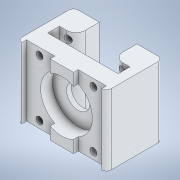
# Autodesk Inventor part: Tensor
Saved by Autodesk Inventor 2021 (Build 250183000, 183)
## iProperties
Created: 2022-10-27
Part Number: Tensor
Material: Generic
Document SubType Name: Modeling
Designer: USUARIO
Density: 1 g/cm^3
Appearance: White
Author: USUARIO
Autodesk Inventor part; units mm, degrees
ref_plane "YZ Plane" through (0, 0, 0) normal (1, 0, 0) x (0, 1, 0)
ref_plane "XZ Plane" through (0, 0, 0) normal (0, 1, 0) x (-1, 0, 0)
ref_plane "XY Plane" through (0, 0, 0) normal (0, 0, 1) x (1, 0, 0)
sketch "Sketch1" plane through (0, 0, 0) normal (0, 1, 0) x (-1, 0, 0)
  line L0 (0, -37.4557) -> (0, 23.9689) construction
  line L1 (8, -2) -> (8, -12)
  line L2 (8, -12) -> (19, -12)
  line L3 (19, -12) -> (19, 12)
  line L4 (19, 12) -> (2, 12)
  line L5 (8, -2) -> (15, -2)
  line L6 (15, -2) -> (15, 3)
  line L7 (15, 3) -> (0, 3)
  line L8 (0, -49.7407) -> (0, 36.2538) projected
  line L9 (-8, -2) -> (-8, -12)
  line L10 (-8, -12) -> (-19, -12)
  line L11 (-19, -12) -> (-19, 12)
  line L12 (-19, 12) -> (2, 12)
  line L13 (-8, -2) -> (-15, -2)
  line L14 (-15, -2) -> (-15, 3)
  line L15 (-15, 3) -> (0, 3)
  line L16 (26.6, 0) -> (-26.6, 0) projected
  point P0 (19, 0)
  point P1 (-19, 0)
  dimension "d12" = 15
  dimension "d13" = 5
  dimension "d14" = 7
  dimension "d15" = 10
  dimension "d16" = 11
  dimension "d18" = 9
  dimension "d19" = 17
  constraints: 30 end point, 7 symmetric about line, 3 parallel, 2 perpendicular, 2 point on line, 2 vertical, 1 collinear, 1 horizontal, 1 midpoint
  measures "d12" distance of L6.end L7.end
  measures "d13" distance of L5.end L6.end
  measures "d14" distance of L1.start L5.end
  measures "d15" distance of L1.start L1.end
  measures "d16" distance of L1.end L2.end
  measures "d18" distance between parallel lines of L4 L7
  measures "d19" distance of L3.end L4.end
extrude "Extrusion1" add sketch "Sketch1" along normal blind 30 contours L5 L6 L16 L3 L2 L1 | L6 L7 L8 L12 L4 L3 L16 | L15 L14 L16 L11 L12 L8 | L14 L13 L9 L10 L11 L16
fillet "Fillet1" radius 4 2 edges at (-8, 15, -2) (8, 15, -2)
sketch "Sketch2" plane through (-19, 0, 12) normal (0, 0, 1) x (1, 0, 0)
  line L0 (0, 0) -> (38, 0) projected
  line L1 (38, 0) -> (38, 30) projected
  line L2 (0, 30) -> (38, 30) projected
  line L3 (0, 0) -> (0, 30) projected
  line L4 (38, 0) -> (38, 30) projected
  line L5 (38, 15) -> (0, 15) construction
  line L6 (0, 0) -> (0, 30) projected
  circle A0 centre (19, 15) radius 11
  circle A1 centre (19, 15) radius 5
  line L7 (0, 0) -> (38, 0) projected
  line L8 (7, 30) -> (7, 0) projected
  line L9 (4, 30) -> (7, 30) projected
  line L10 (4, 0) -> (4, 30) projected
  line L11 (4, 0) -> (7, 0) projected
  line L12 (31, 0) -> (31, 30) projected
  line L13 (31, 0) -> (34, 0) projected
  line L14 (34, 0) -> (34, 30) projected
  line L15 (31, 30) -> (34, 30) projected
  circle A2 centre (30.5, 27) radius 1.5
  line L16 (19, 15) -> (19, 38.5815) construction
  circle A3 centre (7.5, 27) radius 1.5
  circle A4 centre (30.5, 3) radius 1.5
  circle A5 centre (7.5, 3) radius 1.5
  point P0 (19, 0)
  dimension "d23" = 22
  dimension "d24" = 10
  dimension "d25" = 3
  dimension "d26" = 11.5
  dimension "d27" = 12
  constraints: 6 centre point, 4 end point, 3 midpoint, 3 symmetric about line, 1 coincident, 1 vertical, 3 other
  measures "d23" diameter of A0
  measures "d24" diameter of A1
  measures "d25" diameter of A2
  measures "d26" horizontal distance of A0.centre A2.centre
  measures "d27" vertical distance of A2.centre A0.centre
extrude "Extrusion2" cut sketch "Sketch2" against normal blind 7 contours A0
extrude "Extrusion3" cut sketch "Sketch2" against normal through all contours A5 L8 | L8 A5 | A4 L12 | L12 A4 | A3 L8 | L8 A3 | A2 L12 | L12 A2 | A1
fillet "Fillet2" radius 2 4 edges at (19, 15, 12) (-19, 15, 12) (-19, 15, -12) (19, 15, -12)
sketch "Boceto4" plane through (-17, 0, 12) normal (0, 0, 1) x (1, 0, 0)
  circle A0 centre (17, 15) radius 5 projected
  line L0 (0, 0) -> (0, 30) projected
  line L1 (34, 30) -> (34, 0) projected
  line L2 (0, 0) -> (34, 0) projected
  line L3 (32, 30) -> (2, 30) projected
  line L4 (12, 30) -> (12, 24.798)
  circle A1 centre (17, 15) radius 11 projected
  line L5 (22, 30) -> (22, 24.798)
  circle A2 centre (17, 15) radius 5 construction
  line L6 (17, 15) -> (17, 30) construction
  line L7 (32, 0) -> (2, 0) construction
  line L8 (12, 0) -> (12, 5.202)
  line L9 (22, 0) -> (22, 5.202)
  circle A3 centre (17, 15) radius 11 projected
  line L10 (0, 30) -> (34, 30) projected
  circle A4 centre (5.5, 3) radius 1.5 projected
  circle A5 centre (28.5, 27) radius 1.5 projected
  circle A6 centre (5.5, 27) radius 1.5 projected
  circle A7 centre (28.5, 3) radius 1.5 projected
  line L11 (0, 0) -> (0, 30) projected
  line L12 (0, 0) -> (34, 0) projected
  line L13 (34, 30) -> (34, 0) projected
  line L14 (0, 30) -> (34, 30) projected
  circle A8 centre (17, 15) radius 11 projected
  circle A9 centre (28.5, 27) radius 1.5 projected
  circle A10 centre (5.5, 3) radius 1.5 projected
  circle A11 centre (28.5, 3) radius 1.5 projected
  point P0 (17, 0)
  dimension "d44" = 5
  dimension "d45" = 5
  constraints: 10 end point, 4 point on circle, 4 point on line, 4 vertical, 2 collinear, 1 midpoint
  measures "d44" distance between parallel lines of L6 L4
  measures "d45" distance between parallel lines of L6 L5
extrude "Extrusión5" cut sketch "Boceto4" against normal blind 2 contours L0 L10 L3 L4 A1 L8 L2 | L9 A1 L5 L3 L10 L1 L2
equation "\"d45\" = d44"
body "Solid1"
